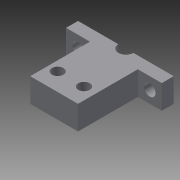
# Autodesk Inventor part: clip_to_shaft_holder(2)
Saved by Autodesk Inventor 2015 (Build 190159000, 159)
## iProperties
Created: 2017-09-27
Part Number: clip_to_shaft_holder(2)
Material: Generic
Document SubType Name: Modeling
Designer: Anshul
Density: 1 g/cm^3
Appearance: Default
Author: Anshul
Autodesk Inventor part; units mm, degrees
ref_plane "YZ Plane" through (0, 0, 0) normal (1, 0, 0) x (0, 1, 0)
ref_plane "XZ Plane" through (0, 0, 0) normal (0, 1, 0) x (-1, 0, 0)
ref_plane "XY Plane" through (0, 0, 0) normal (0, 0, 1) x (1, 0, 0)
sketch "Sketch1" plane through (0, 0, 0) normal (0, 1, 0) x (-1, 0, 0)
  circle A0 centre (0, 0) radius 3.15
  line L0 (10, 5) -> (10, 30)
  line L1 (10, 30) -> (-10, 30)
  line L2 (-10, 30) -> (-10, 5)
  line L3 (10, -5) -> (10, -30)
  line L4 (10, -30) -> (-10, -30)
  line L5 (-10, -30) -> (-10, -5)
  line L6 (-10, 30) -> (-10, 15)
  line L7 (10, 30) -> (10, 15)
  line L8 (10, -30) -> (10, -15)
  line L9 (-10, -15) -> (-10, -30)
  line L10 (2.5151, -1.8965) -> (-2.5151, -1.8965)
  circle A1 centre (0, 0) radius 4.5
  line L11 (10, 0) -> (3.15, 0)
  line L12 (-3.15, 0) -> (-10, 0)
  line L13 (-10, 0) -> (-20, 0)
  line L14 (-20, 0) -> (-20, -5)
  line L15 (-20, -5) -> (-10, -5)
  line L16 (10, 0) -> (20, 0)
  line L17 (20, 0) -> (20, -5)
  line L18 (20, -5) -> (10, -5)
  line L19 (-4.5, 0) -> (-3.15, 0)
  line L20 (3.15, 0) -> (4.5, 0)
  line L21 (20, 0) -> (20, 5)
  line L22 (20, 5) -> (10, 5)
  line L23 (-20, 0) -> (-20, 5)
  line L24 (-20, 5) -> (-10, 5)
  circle A2 centre (-5, 22.5) radius 2.25
  circle A3 centre (6, 22.5) radius 2.25
  circle A4 centre (-6, -22.5) radius 2.25
  circle A5 centre (6, -22.5) radius 2.25
  circle A6 centre (-5, 22.5) radius 2.4
  circle A7 centre (6, 22.5) radius 2.4
  dimension "d0" = 6.3
  dimension "d6" = 15
  dimension "d34" = 9
  dimension "d35" = 10
  dimension "d36" = 5
  dimension "d37" = 10
  dimension "d38" = 5
  dimension "d43" = 5
  dimension "d44" = 5
  dimension "d45" = 4.5
  dimension "d46" = 4.5
  dimension "d47" = 4.5
  dimension "d48" = 4.5
  dimension "d61" = 4.8
  dimension "d62" = 4.8
  constraints: 50 end point, 11 perpendicular, 10 point on line, 8 centre point, 6 point on circle, 4 coincident, 3 collinear, 2 horizontal, 2 vertical
  measures "d0" diameter of A0
  measures "d6" distance of L1.end L6.end
  measures "d34" diameter of A1
  measures "d35" distance of L12.end L13.end
  measures "d36" distance of L13.end L14.end
  measures "d37" distance of L11.start L16.end
  measures "d38" distance of L16.end L17.end
  measures "d43" distance of L16.end L21.end
  measures "d44" distance of L13.end L23.end
  measures "d45" diameter of A2
  measures "d46" diameter of A3
  measures "d47" diameter of A4
  measures "d48" diameter of A5
  measures "d61" diameter of A6
  measures "d62" diameter of A7
extrude "Extrusion10" add sketch "Sketch1" along normal blind 10 contours A0 L12 A1 L11 | A1 L12 L13 L23 L24 L2 L1 L0 L22 L21 L16 L11 | A6 | A7 picked at (-4.0064, 0.359)
extrude "Extrusion11" add sketch "Sketch1" against normal blind 5 contours A0 L12 A1 L11 picked at (-4.0064, 0.359)
sketch "Sketch3" plane through (-3.15, 10, 0) normal (0, 0, -1) x (-1, 0, 0)
  line L0 (-23.15, -10) -> (-23.15, -5)
  line L1 (-23.15, -10) -> (-23.15, 0) projected
  line L2 (-23.15, -5) -> (-18.15, -5)
  line L3 (16.85, -10) -> (16.85, -5)
  line L4 (16.85, -10) -> (16.85, 0) projected
  line L5 (16.85, -5) -> (11.85, -5)
  circle A0 centre (-18.15, -5) radius 2.35
  circle A1 centre (11.85, -5) radius 2.35
  circle A2 centre (-18.15, -5) radius 2.4
  circle A3 centre (11.85, -5) radius 2.4
  point P0 (-3.15, -10)
  dimension "d53" = 5
  dimension "d54" = 5
  dimension "d55" = 5
  dimension "d56" = 5
  dimension "d57" = 4.7
  dimension "d58" = 4.7
  dimension "d65" = 4.8
  dimension "d66" = 4.8
  constraints: 8 end point, 4 centre point, 4 coincident, 2 midpoint, 1 perpendicular, 1 point on line
  measures "d53" distance of L0.start L0.end
  measures "d54" distance of L0.end L2.end
  measures "d55" distance of L3.start L3.end
  measures "d56" distance of L3.end L5.end
  measures "d57" diameter of A0
  measures "d58" diameter of A1
  measures "d65" diameter of A2
  measures "d66" diameter of A3
extrude "Extrusion13" cut sketch "Sketch1" along normal blind 10 contours A6 | A7
extrude "Extrusion14" cut sketch "Sketch3" against normal blind 10 contours A0 | A2 | A1 | A3
body "Solid3"
